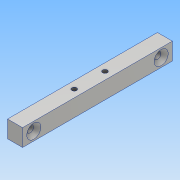
# Autodesk Inventor part: Pancake_Flexi Pipe Mount
Saved by Autodesk Inventor 2018.1 (Build 221171000, 171)
## iProperties
Created: 2019-02-26
Part Number: Pancake_Flexi Pipe Mount
Material: Aluminum 6061
Document SubType Name: Modeling
Designer: James
Density: 2.7 g/cm^3
Appearance: Aluminum - Flat
Author: James
Autodesk Inventor part; units mm, degrees
ref_plane "YZ Plane" through (0, 0, 0) normal (1, 0, 0) x (0, 1, 0)
ref_plane "XZ Plane" through (0, 0, 0) normal (0, 1, 0) x (-1, 0, 0)
ref_plane "XY Plane" through (0, 0, 0) normal (0, 0, 1) x (1, 0, 0)
sketch "Sketch1" plane through (0, 0, 0) normal (0, 0, 1) x (1, 0, 0)
  line L0 (0, 0) -> (10, 0)
  line L1 (10, 0) -> (10, 100)
  line L2 (10, 100) -> (0, 100)
  line L3 (0, 100) -> (0, 0)
  dimension "d0" = 10
  dimension "d1" = 100
  constraints: 8 end point, 2 parallel, 1 horizontal, 1 perpendicular
  measures "d0" distance of L0.start L0.end
  measures "d1" distance of L0.end L1.end
extrude "Extrusion1" add sketch "Sketch1" along normal blind 11.5
sketch "Sketch2" plane through (0, 0, 11.5) normal (0, 0, 1) x (1, 0, 0)
  line L0 (10, 100) -> (0, 100) projected
  line L1 (0, 0) -> (10, 0) projected
  point P0 (5, 39.5)
  point P1 (5, 60)
  point P2 (5, 100)
  dimension "d4" = 20.5
  dimension "d5" = 40
  dimension "d14" = 39.5
  dimension "d24" = 100
  constraints: 2 vertical alignment, 1 midpoint
  measures "d4" distance of point (5, 39.5) point (5, 60)
  measures "d5" distance from line of L0 point (5, 60)
  measures "d14" distance from line of L1 point (5, 39.5)
  measures "d24" distance between parallel lines of L1 L0
hole "Hole1" at (5, 39.5, 11.5) at (5, 60, 11.5) direction (0, 0, -1) diameter 3.242 end through all thread size "M4x0.7" class "6H" standard "ANSI Metric M Profile"
sketch "Sketch3" plane through (10, 0, 0) normal (1, 0, 0) x (0, 0, -1)
  line L0 (0, 100) -> (-11.5, 100) projected
  line L1 (0, 0) -> (-11.5, 0) projected
  point P0 (-5.75, 92.5)
  point P1 (-5.75, 7.5)
  point P2 (-5.75, 100)
  dimension "d15" = 7.5
  dimension "d16" = 7.5
  constraints: 2 vertical alignment, 1 midpoint
  measures "d15" distance from line of point (-5.75, 92.5) L0
  measures "d16" distance from line of L1 point (-5.75, 7.5)
hole "Hole2" at (10, 92.5, 5.75) at (10, 7.5, 5.75) direction (-1, 0, 0) diameter 4.5 end through all countersink diameter 9.4 countersink angle 90 clearance for "Flat Head Machine Screw" size "M4" standard "Ansi Metric M Profile"
equation "\"d16\" = d15"
body "Solid1"
